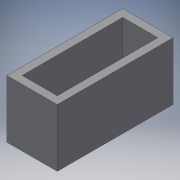
# Autodesk Inventor part: batteryholder
Saved by Autodesk Inventor 2018.2 (Build 222227000, 227)
## iProperties
Created: 2019-04-15
Part Number: batteryholder
Material: Generic
Vendor: HHMI: JRC - ID&F
Document SubType Name: Modeling
Designer: sawtelles
Density: 1 g/cm^3
Appearance: Default
RuleStatus: InUse
AfterDocSave0: file://Part Number Cleaner
Author: sawtelles
Revision Number: 0
DESIGN DEPARTMENT: HHMI: JRC - ID&F
ALTERED ITEM PART NUMBER: N/A
ALTERED ITEM VENDOR: N/A
ALTERED ITEM DESCRIPTION: N/A
Autodesk Inventor part; units mm, degrees
ref_plane "YZ Plane" through (0, 0, 0) normal (1, 0, 0) x (0, 1, 0)
ref_plane "XZ Plane" through (0, 0, 0) normal (0, 1, 0) x (-1, 0, 0)
ref_plane "XY Plane" through (0, 0, 0) normal (0, 0, 1) x (1, 0, 0)
sketch "Sketch1" plane through (0, 0, 0) normal (0, 1, 0) x (-1, 0, 0)
  line L0 (0, 0) -> (25.4, 0)
  line L1 (25.4, 0) -> (25.4, -58.42)
  line L2 (25.4, -58.42) -> (0, -58.42)
  line L3 (0, -58.42) -> (0, 0)
  dimension "d0" = 25.4
  dimension "d1" = 58.42
  constraints: 8 end point, 2 parallel, 1 horizontal, 1 perpendicular
  measures "d0" distance of L1.end L2.end
  measures "d1" distance of L0.end L1.end
extrude "Extrusion1" add sketch "Sketch1" along normal blind 3.81
sketch "Sketch2" plane through (0, 3.81, 0) normal (0, 1, 0) x (1, 0, 0)
  line L0 (-3.81, 3.81) -> (-21.59, 3.81)
  line L1 (-21.59, 3.81) -> (-21.59, 54.61)
  line L2 (-21.59, 54.61) -> (-3.81, 54.61)
  line L3 (-3.81, 54.61) -> (-3.81, 3.81)
  line L4 (-25.4, 58.42) -> (-25.4, 0) projected
  line L5 (-25.4, 0) -> (0, 0) projected
  line L6 (0, 0) -> (0, 58.42) projected
  line L7 (0, 58.42) -> (-25.4, 58.42) projected
  dimension "d4" = 17.78
  dimension "d5" = 50.8
  constraints: 8 end point, 2 parallel, 1 horizontal, 1 perpendicular
  measures "d4" distance of L1.end L2.end
  measures "d5" distance of L0.end L1.end
extrude "Extrusion2" add sketch "Sketch2" along normal blind 25.4
sketch "Sketch3" plane through (0, 3.81, 0) normal (0, 1, 0) x (1, 0, 0)
  point P0 (0, 0)
  point P1 (-12.7, 16.51)
  point P2 (-12.7, 41.91)
hole "Hole1" at (-12.7, 3.81, -16.51) at (-12.7, 3.81, -41.91) direction (0, -1, 0) diameter 6.35 end through all countersink diameter 12.065 countersink angle 82
body "Solid1"
